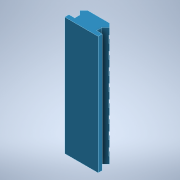
# Autodesk Inventor part: Rail
Saved by Autodesk Inventor 2022 (Build 260153000, 153)
## iProperties
Created: 2023-08-28
Part Number: Rail
Material: Типовые
Document SubType Name: Modeling
Designer: user
Density: 1 g/cm^3
Appearance: По умолчанию
Author: user
## iProperties of the stored document Rail_3DПЕЧАТЬ.ipt
Created: 2023-08-30
Part Number: Rail_3DПЕЧАТЬ
Material: Типовые
Document SubType Name: Modeling
Designer: user
Density: 1 g/cm^3
Appearance: По умолчанию
Author: user
Autodesk Inventor part; units mm, degrees
ref_plane "YZ Plane" through (0, 0, 0) normal (1, 0, 0) x (0, 1, 0)
ref_plane "XZ Plane" through (0, 0, 0) normal (0, 1, 0) x (-1, 0, 0)
ref_plane "XY Plane" through (0, 0, 0) normal (0, 0, 1) x (1, 0, 0)
sketch "Эскиз1" plane through (0, 0, 0) normal (0, 1, 0) x (-1, 0, 0)
  line L0 (-49.8359, -27.3218) -> (-34.1641, -27.3218)
  line L1 (-34.1641, -27.3218) -> (-31.3955, -24.5532)
  line L2 (-31.3955, -24.5532) -> (-31.3955, -24.5024)
  line L3 (-31.3955, -24.5024) -> (-34.1641, -21.7338)
  line L4 (-34.1641, -21.7338) -> (-34.1641, -18)
  line L5 (-34.1641, -18) -> (-30, -18)
  line L6 (-30, -18) -> (-30, -15)
  line L7 (-30, -15) -> (-54, -15)
  line L8 (-54, -15) -> (-54, -18)
  line L9 (-54, -18) -> (-49.8359, -18)
  line L10 (-49.8359, -18) -> (-49.8359, -21.7338)
  line L11 (-49.8359, -21.7338) -> (-52.6045, -24.5024)
  line L12 (-52.6045, -24.5024) -> (-52.6045, -24.5532)
  line L13 (-52.6045, -24.5532) -> (-49.8359, -27.3218)
  line L14 (-56.1832, -23.1562) -> (-23.3808, -23.1562) construction
  line L15 (-55.8733, -25.8994) -> (-24.0699, -25.8994) construction
  line L16 (-55.8733, -24.5278) -> (-24.0699, -24.5278) construction
  line L17 (-25.0606, -25.8994) -> (-25.0606, -24.5278) construction
  line L18 (-26.6052, -24.5278) -> (-26.6052, -23.1562) construction
  line L19 (-37.1641, -27.3218) -> (-38.6641, -24.3218)
  line L20 (-38.6641, -24.3218) -> (-45.3359, -24.3218)
  line L21 (-45.3359, -24.3218) -> (-46.8359, -27.3218)
  point P0 (0, 0)
  point P1 (-31.3955, -24.5278)
  dimension "d0" = 21.209
  dimension "d1" = 9.3218
  dimension "d2" = 15.6718
  dimension "d3" = 4.1656
  dimension "d4" = 2.7432
  dimension "d5" = 45
  dimension "d6" = 45
  dimension "d7" = 45
  dimension "d8" = 3
  dimension "d9" = 24
  dimension "d10" = 15
  dimension "d11" = 30
  dimension "d23" = 3
  dimension "d24" = 3
  dimension "d25" = 1.5
  dimension "d26" = 1.5
  dimension "d27" = 3
  constraints: 44 end point, 9 point on line, 8 perpendicular, 7 equal length, 5 horizontal, 3 parallel, 1 midpoint
  measures "d0" distance between parallel lines of L2 L12
  measures "d1" distance between parallel lines of L5 L0
  measures "d2" distance between parallel lines of L4 L10
  measures "d3" distance between parallel lines of L14 L0
  measures "d4" distance between parallel lines of L15 L14
  measures "d5" angle of L13 L15
  measures "d6" angle of L15 L11
  measures "d7" angle of L15 L3
  measures "d8" distance between parallel lines of L7 L5
  measures "d9" distance between parallel lines of L8 L6
  measures "d10" distance from line of point (0, 0) L7
  measures "d11" distance from line of point (0, 0) L6
  measures "d23" distance of L21.end L0.start
  measures "d24" distance of L19.start L0.end
  measures "d25" horizontal distance of L19.start L19.end
  measures "d26" horizontal distance of L21.end L20.end
  measures "d27" distance between parallel lines of L0 L20
extrude "Выдавливание1" add sketch "Эскиз1" along normal mid plane 85
sketch "Эскиз2" plane through (54, -42.5, -18) normal (1, 0, 0) x (0, 0, -1)
  line L0 (9.3218, 85) -> (6.5532, 85) projected
  line L1 (6.3218, 85) -> (6.3218, 0)
  line L2 (6.5532, 0) -> (9.3218, 0) projected
  line L3 (9.3218, 85) -> (9.3218, 0) projected
  line L4 (9.3218, 0) -> (9.3218, 85) projected
  line L5 (9.3218, 80.2324) -> (6.3218, 80.2324)
  line L6 (9.3218, 75) -> (6.3218, 75)
  point P0 (-18, 42.5)
  dimension "d14" = 3
  dimension "d15" = 5.2324
  dimension "d16" = 10
  constraints: 6 end point, 6 point on line, 2 perpendicular, 1 vertical
  measures "d14" distance between parallel lines of L1 L3
  measures "d15" distance between parallel lines of L6 L5
  measures "d16" distance between parallel lines of L0 L6
extrude "Выдавливание2" cut sketch "Эскиз2" against normal through all
pattern_linear "Прямоуг.массив1" count 8 spacing 10 along (0, -1, 0) of "Выдавливание2"
equation "\"d24\" = d23"
equation "\"d26\" = d25"
